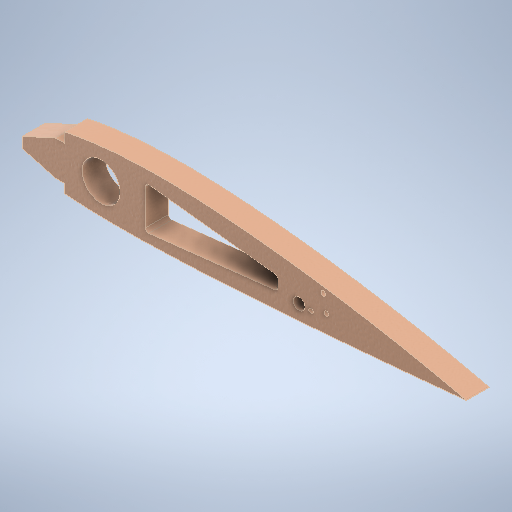
# Autodesk Inventor part: 2414 basic aerofoil
Saved by Autodesk Inventor 2025.1 (Build 291241000, 241)
## iProperties
Created: 2024-11-04
Part Number: 2414 basic aerofoil
Material: Polyurethane Foam
Document SubType Name: Modeling
Designer: johan
Density: 0.032 g/cm^3
Appearance: Coarse Textured - Umber
Author: johan
Autodesk Inventor part; units mm, degrees
ref_plane "YZ Plane" through (0, 0, 0) normal (1, 0, 0) x (0, 1, 0)
ref_plane "XZ Plane" through (0, 0, 0) normal (0, 1, 0) x (-1, 0, 0)
ref_plane "XY Plane" through (0, 0, 0) normal (0, 0, 1) x (1, 0, 0)
sketch "Sketch2" plane through (0, 0, 0) normal (0, 0, 1) x (1, 0, 0)
  spline S0 degree 5 poles (319.5633, 0.0573) (319.5622, 0.0645) (319.5873, 0.0852) (319.7357, 0.1422) (318.5514, 0.0989) (319.5116, 0.3205) (317.7694, 0.3117) (318.0865, 0.563) (316.6439, 0.6855) (316.0954, 0.948) (314.7794, 1.1779) (313.6787, 1.4773) (312.2394, 1.7863) (310.766, 2.136) (309.0996, 2.5093) (307.3242, 2.9134) (305.3998, 3.342) (303.349, 3.7975) (301.1634, 4.2757) (298.8504, 4.7782) (296.4091, 5.301) (293.8432, 5.8446) (291.1548, 6.4061) (288.3466, 6.9857) (285.4207, 7.5803) (282.3807, 8.1894) (279.2284, 8.8107) (275.968, 9.4437) (272.6016, 10.0865) (269.1329, 10.7361) (265.5656, 11.3942) (261.9019, 12.0551) (258.1469, 12.7207) (254.3029, 13.3883) (250.3742, 14.0555) (246.3647, 14.7217) (242.2776, 15.3854) (238.118, 16.0441) (233.8887, 16.6979) (229.5952, 17.3434) (225.2402, 17.981) (220.8297, 18.6074) (216.3658, 19.2226) (211.8552, 19.8242) (207.3009, 20.4107) (202.7077, 20.9813) (198.0804, 21.5339) (193.4232, 22.0679) (188.7413, 22.58) (184.0389, 23.0713) (179.321, 23.5382) (174.592, 23.982) (169.8567, 24.3971) (165.1201, 24.7874) (160.3872, 25.1472) (155.6604, 25.4776) (150.948, 25.7772) (146.2454, 26.0449) (141.5744, 26.278) (136.9015, 26.4795) (132.2479, 26.6311) (127.6319, 26.7393) (123.054, 26.7999) (118.5202, 26.8147) (114.0397, 26.7815) (109.6094, 26.7031) (105.2517, 26.5723) (100.9331, 26.4088) (96.7495, 26.1663) (92.5147, 25.9483) (88.6376, 25.5343) (84.2302, 25.3974) (81.2071, 24.5612) (76.5297, 24.5259) (73.18, 23.8676) (69.3619, 23.413) (65.9721, 22.8018) (62.3454, 22.244) (59.4319, 21.514) (55.4307, 21.0148) (53.2464, 20.1084) (49.5889, 19.537) (47.2944, 18.6473) (44.3884, 17.909) (41.914, 17.071) (39.4431, 16.2394) (37.1538, 15.3738) (34.9769, 14.4941) (32.9455, 13.5944) (31.0501, 12.6807) (29.296, 11.7542) (27.6838, 10.8151) (26.2147, 9.8673) (24.8899, 8.9103) (23.7091, 7.9466) (22.6766, 6.9761) (21.7838, 6.0003) (21.0519, 5.0188) (20.4402, 4.0317) (20.0369, 3.0394) (19.6679, 2.0412) (19.7059, 1.0482) (19.3667, 0.0428) (19.9014, -0.9137) (20.0594, -1.8759) (20.6154, -2.7916) (21.2041, -3.6802) (21.9915, -4.5317) (22.8926, -5.3516) (23.9468, -6.1384) (25.1324, -6.8944) (26.4586, -7.6188) (27.9182, -8.3124) (29.5137, -8.9751) (31.2408, -9.6071) (33.0997, -10.2067) (35.0892, -10.7758) (37.2002, -11.3131) (39.4562, -11.8174) (41.7927, -12.2939) (44.3651, -12.7275) (46.7744, -13.1584) (50.0005, -13.481) (52.1533, -13.8927) (55.9371, -14.1294) (58.2153, -14.4717) (61.732, -14.6854) (64.8012, -14.9153) (68.2287, -15.092) (71.6338, -15.2498) (75.1915, -15.3722) (78.8138, -15.4692) (82.5326, -15.5359) (86.3291, -15.5764) (90.2061, -15.5901) (94.1575, -15.5787) (98.1812, -15.5438) (102.2727, -15.4851) (106.4286, -15.4059) (110.6456, -15.3062) (114.9188, -15.1867) (119.2459, -15.0512) (123.6218, -14.8988) (128.0442, -14.7319) (132.5111, -14.552) (137.0141, -14.3592) (141.5621, -14.1606) (146.1675, -13.9403) (150.787, -13.7052) (155.434, -13.4523) (160.0951, -13.1857) (164.7676, -12.9046) (169.4465, -12.6129) (174.1261, -12.3082) (178.8033, -11.9955) (183.4722, -11.6727) (188.1294, -11.3426) (192.7696, -11.0072) (197.3886, -10.6641) (201.9818, -10.3188) (206.5448, -9.9678) (211.0728, -9.6157) (215.5623, -9.2611) (220.0069, -8.9047) (224.4048, -8.5497) (228.7492, -8.193) (233.0373, -7.8393) (237.2647, -7.4865) (241.4259, -7.1353) (245.5189, -6.7884) (249.5374, -6.4441) (253.4791, -6.104) (257.3389, -5.7683) (261.1136, -5.4376) (264.7987, -5.113) (268.3914, -4.7937) (271.8871, -4.4807) (275.2826, -4.1749) (278.5752, -3.8759) (281.7596, -3.585) (284.8354, -3.3021) (287.7962, -3.0278) (290.6419, -2.763) (293.3673, -2.5063) (295.9711, -2.2616) (298.4499, -2.0246) (300.8007, -1.801) (303.0232, -1.5859) (305.1102, -1.385) (307.0698, -1.1939) (308.8781, -1.0169) (310.5784, -0.8499) (312.0781, -0.7003) (313.5527, -0.5569) (314.6651, -0.4406) (316.0303, -0.3144) (316.5535, -0.2432) (318.0889, -0.1199) (317.6732, -0.1146) (319.5611, 0.0154) (318.488, -0.03) (319.7124, 0.0524) (319.5915, 0.0431) (319.5644, 0.0506) (319.5633, 0.0573) knots 0 0 0 0 0 0 0.001187 0.002346 0.003989 0.006081 0.008474 0.011129 0.014019 0.017125 0.020431 0.023922 0.027589 0.03142 0.035408 0.039543 0.04382 0.048231 0.05277 0.057431 0.062209 0.067099 0.072096 0.077195 0.082391 0.087681 0.09306 0.098523 0.104068 0.10969 0.115384 0.121149 0.126979 0.132871 0.138822 0.144829 0.150887 0.156993 0.163144 0.169337 0.175568 0.181834 0.188131 0.194457 0.200808 0.207181 0.213572 0.219979 0.226398 0.232826 0.239259 0.245695 0.252131 0.258563 0.264988 0.271403 0.277808 0.284202 0.290583 0.296947 0.303291 0.309608 0.315893 0.322143 0.328354 0.334523 0.340648 0.346723 0.352747 0.358657 0.364567 0.370414 0.376198 0.381913 0.387616 0.393187 0.398728 0.404136 0.40949 0.414723 0.419864 0.42486 0.429808 0.434623 0.439363 0.443992 0.448508 0.452906 0.457184 0.461338 0.465365 0.469264 0.473032 0.47667 0.480179 0.483564 0.486831 0.489993 0.493064 0.496069 0.499033 0.501972 0.504912 0.507875 0.510883 0.513952 0.517109 0.52037 0.523745 0.527242 0.530864 0.534612 0.538487 0.542486 0.546608 0.55085 0.555208 0.559679 0.564259 0.568979 0.573768 0.578707 0.583689 0.588762 0.59389 0.599137 0.604414 0.609823 0.615307 0.620863 0.626488 0.632178 0.63793 0.643742 0.64961 0.655531 0.661502 0.667521 0.673583 0.679687 0.685829 0.692006 0.698215 0.704456 0.710729 0.717031 0.723359 0.72971 0.736079 0.742458 0.748845 0.755237 0.76163 0.768021 0.774408 0.780786 0.787154 0.793507 0.799843 0.806158 0.812449 0.818713 0.824947 0.831148 0.837311 0.843434 0.849514 0.855546 0.861529 0.867457 0.873328 0.879138 0.884884 0.890561 0.896166 0.901696 0.907146 0.912512 0.91779 0.922975 0.928065 0.933053 0.937935 0.942706 0.947361 0.951895 0.956301 0.960574 0.964706 0.968691 0.97252 0.976185 0.979675 0.982979 0.986084 0.988974 0.991629 0.994021 0.996112 0.997735 0.998873 1 1 1 1 1 1
  circle A0 centre (79.5135, 4.5678) radius 12.4155
  line L0 (79.5135, 4.5678) -> (79.5135, 24.6083) construction
  circle A1 centre (209.5633, 0.0573) radius 3.786
  line L1 (319.5633, 0.0573) -> (219.5633, 0.0573) construction
  line L2 (27.919, 4.5057) -> (27.919, -2.4943)
  line L3 (19.627, 1.0326) -> (319.5633, 0.0573) construction
  line L4 (49.7105, 14.4213) -> (55.6079, 14.4213)
  line L5 (49.7104, -8.4915) -> (55.6078, -8.4915)
  line L6 (27.919, 4.5057) -> (49.7105, 14.4213)
  line L7 (27.919, -2.4943) -> (49.7104, -8.4915)
  line L8 (55.6079, 14.4213) -> (55.6079, 20.8726)
  line L9 (55.6078, -8.4915) -> (55.6078, -14.1513)
  line L10 (108.6496, 16.3299) -> (108.6496, -7.1942)
  line L11 (110.8735, -9.1817) -> (193.8736, 0.1678)
  line L12 (195.6498, 2.1552) -> (195.6498, 6.9805)
  line L13 (193.8736, 8.9679) -> (110.8735, 18.3173)
  arc A2 (110.8735, 18.3173) -> (108.6496, 16.3299) centre (110.6496, 16.3299) ccw
  arc A3 (108.6496, -7.1942) -> (110.8735, -9.1817) centre (110.6496, -7.1942) ccw
  arc A4 (193.8736, 0.1678) -> (195.6498, 2.1552) centre (193.6498, 2.1552) ccw
  arc A5 (195.6498, 6.9805) -> (193.8736, 8.9679) centre (193.6498, 6.9805) ccw
  circle A6 centre (227.5633, 3.4733) radius 1.5
  circle A7 centre (217.5082, 0.0573) radius 1.5
  circle A8 centre (225.5082, 13.9137) radius 1.5
  line L14 (227.5633, 3.4733) -> (254.2882, 3.4733) construction
  line L15 (227.5633, 3.4733) -> (184.262, 28.4733) construction
  line L16 (217.5082, 0.0573) -> (225.5082, 13.9137) construction
  point P0 (0, 0)
  point P1 (319.3573, 0.1272)
  point P2 (318.9918, 0.2142)
  point P3 (318.4802, 0.3354)
  point P4 (317.8238, 0.4911)
  point P5 (317.0222, 0.6801)
  point P6 (316.0769, 0.9024)
  point P7 (314.9885, 1.1568)
  point P8 (313.7582, 1.443)
  point P9 (312.3866, 1.7598)
  point P10 (310.8752, 2.1063)
  point P11 (309.2258, 2.4819)
  point P12 (307.4393, 2.8854)
  point P13 (305.5178, 3.3153)
  point P14 (303.4628, 3.7707)
  point P15 (301.2764, 4.2501)
  point P16 (298.9607, 4.7526)
  point P17 (296.5175, 5.2764)
  point P18 (293.9492, 5.8203)
  point P19 (291.2585, 6.3828)
  point P20 (288.4478, 6.9627)
  point P21 (285.5195, 7.5582)
  point P22 (282.4766, 8.1678)
  point P23 (279.3218, 8.79)
  point P24 (276.0584, 9.4236)
  point P25 (272.6891, 10.0668)
  point P26 (269.2175, 10.7178)
  point P27 (265.6469, 11.3757)
  point P28 (261.9803, 12.0381)
  point P29 (258.2219, 12.7041)
  point P30 (254.3747, 13.3722)
  point P31 (250.4426, 14.0403)
  point P32 (246.4295, 14.7072)
  point P33 (242.339, 15.3714)
  point P34 (238.1756, 16.0311)
  point P35 (233.9428, 16.6851)
  point P36 (229.6454, 17.3316)
  point P37 (225.2869, 17.9694)
  point P38 (220.8723, 18.5967)
  point P39 (216.4049, 19.2123)
  point P40 (211.8901, 19.8144)
  point P41 (207.332, 20.4015)
  point P42 (202.7347, 20.9724)
  point P43 (198.1034, 21.5256)
  point P44 (193.4423, 22.0596)
  point P45 (188.7563, 22.5726)
  point P46 (184.0499, 23.0637)
  point P47 (179.3279, 23.5314)
  point P48 (174.5948, 23.9745)
  point P49 (169.8554, 24.3909)
  point P50 (165.1148, 24.7803)
  point P51 (160.3775, 25.1406)
  point P52 (155.6479, 25.4709)
  point P53 (150.9316, 25.7703)
  point P54 (146.233, 26.0373)
  point P55 (141.557, 26.2707)
  point P56 (136.882, 26.4681)
  point P57 (132.2209, 26.6211)
  point P58 (127.5964, 26.7282)
  point P59 (123.0133, 26.7888)
  point P60 (118.4761, 26.8026)
  point P61 (113.9902, 26.7693)
  point P62 (109.5601, 26.6886)
  point P63 (105.191, 26.5611)
  point P64 (100.8866, 26.3866)
  point P65 (96.6524, 26.1647)
  point P66 (92.4927, 25.8975)
  point P67 (88.4121, 25.5832)
  point P68 (84.4152, 25.2282)
  point P69 (80.9052, 24.7441)
  point P70 (76.6873, 24.3761)
  point P71 (72.9635, 23.8905)
  point P72 (69.3402, 23.3611)
  point P73 (65.8208, 22.7938)
  point P74 (62.4086, 22.1883)
  point P75 (59.107, 21.5464)
  point P76 (52.8493, 20.1606)
  point P77 (49.7105, 19.4213)
  point P78 (47.0737, 18.6507)
  point P79 (44.3741, 17.8542)
  point P80 (41.8034, 17.0322)
  point P81 (39.3638, 16.1874)
  point P82 (37.0583, 15.3213)
  point P83 (34.8884, 14.4363)
  point P84 (32.8568, 13.534)
  point P85 (30.965, 12.6166)
  point P86 (29.2145, 11.686)
  point P87 (27.6071, 10.7437)
  point P88 (26.1443, 9.7921)
  point P89 (24.8269, 8.8324)
  point P90 (23.6566, 7.8664)
  point P91 (22.6336, 6.8953)
  point P92 (21.7591, 5.9209)
  point P93 (21.0334, 4.9441)
  point P94 (20.4571, 3.9661)
  point P95 (20.0308, 2.9875)
  point P96 (19.7539, 2.0098)
  point P97 (19.5632, 0.0573)
  point P98 (19.8205, -0.9033)
  point P99 (20.1376, -1.8357)
  point P100 (20.6002, -2.7402)
  point P101 (21.208, -3.6159)
  point P102 (21.9598, -4.4628)
  point P103 (22.8544, -5.2806)
  point P104 (23.8909, -6.069)
  point P105 (25.0681, -6.8277)
  point P106 (26.3846, -7.5561)
  point P107 (27.8384, -8.2539)
  point P108 (29.4284, -8.9211)
  point P109 (31.1522, -9.5571)
  point P110 (33.0086, -10.1613)
  point P111 (34.9949, -10.734)
  point P112 (37.1093, -11.2746)
  point P113 (39.3497, -11.7828)
  point P114 (41.7134, -12.2586)
  point P115 (44.198, -12.702)
  point P116 (46.8014, -13.1127)
  point P117 (49.7104, -13.4915)
  point P118 (52.3532, -13.8357)
  point P119 (58.3469, -14.4294)
  point P120 (61.5023, -14.6781)
  point P121 (64.7591, -14.8953)
  point P122 (68.1149, -15.0813)
  point P123 (71.5661, -15.237)
  point P124 (75.1094, -15.3627)
  point P125 (78.7418, -15.4596)
  point P126 (82.46, -15.528)
  point P127 (86.2607, -15.5691)
  point P128 (90.14, -15.5838)
  point P129 (94.0946, -15.5733)
  point P130 (98.1212, -15.5388)
  point P131 (102.2159, -15.4812)
  point P132 (106.3751, -15.4023)
  point P133 (110.5952, -15.303)
  point P134 (114.872, -15.1845)
  point P135 (119.2022, -15.0489)
  point P136 (123.5813, -14.8971)
  point P137 (128.006, -14.7306)
  point P138 (132.4718, -14.5509)
  point P139 (136.9748, -14.3598)
  point P140 (141.5285, -14.1576)
  point P141 (146.1365, -13.9383)
  point P142 (150.7679, -13.7022)
  point P143 (155.4191, -13.4499)
  point P144 (160.0853, -13.1829)
  point P145 (164.7617, -12.9024)
  point P146 (169.4444, -12.6099)
  point P147 (174.1283, -12.306)
  point P148 (178.8092, -11.9925)
  point P149 (183.4823, -11.67)
  point P150 (188.1434, -11.34)
  point P151 (192.7877, -11.0037)
  point P152 (197.4106, -10.6614)
  point P153 (202.0079, -10.3149)
  point P154 (206.5747, -9.9645)
  point P155 (211.1069, -9.6117)
  point P156 (215.5999, -9.2568)
  point P157 (220.0489, -8.9007)
  point P158 (224.4503, -8.5446)
  point P159 (228.7987, -8.1885)
  point P160 (233.0906, -7.8339)
  point P161 (237.3214, -7.4808)
  point P162 (241.4866, -7.1298)
  point P163 (245.5828, -6.7821)
  point P164 (249.6052, -6.4377)
  point P165 (253.5502, -6.0972)
  point P166 (257.4136, -5.7612)
  point P167 (261.1915, -5.4303)
  point P168 (264.88, -5.1051)
  point P169 (268.4758, -4.7856)
  point P170 (271.9747, -4.4724)
  point P171 (275.3734, -4.1661)
  point P172 (278.6686, -3.867)
  point P173 (281.8564, -3.5757)
  point P174 (284.9344, -3.2925)
  point P175 (287.8984, -3.018)
  point P176 (290.7463, -2.7525)
  point P177 (293.4745, -2.4963)
  point P178 (296.0806, -2.2503)
  point P179 (298.5616, -2.0142)
  point P180 (300.9151, -1.7892)
  point P181 (303.1387, -1.575)
  point P182 (305.23, -1.3728)
  point P183 (307.1866, -1.1823)
  point P184 (309.007, -1.0041)
  point P185 (310.6885, -0.8385)
  point P186 (312.2302, -0.6861)
  point P187 (313.6297, -0.5472)
  point P188 (314.8861, -0.4221)
  point P189 (315.9976, -0.3108)
  point P190 (316.9636, -0.2139)
  point P191 (317.7826, -0.1314)
  point P192 (318.4537, -0.0636)
  point P193 (318.9766, -0.0108)
  point P194 (319.3503, 0.027)
  point P195 (319.5743, 0.0498)
  point P196 (27.919, 1.0057)
  point P197 (108.6496, 18.5678)
  point P198 (108.6496, -9.4322)
  point P199 (195.6498, 0.3678)
  dimension "d2" = 300.0001
  dimension "d18" = 7.572
  dimension "d19" = 110
  dimension "d22" = 100
  dimension "d23" = 7
  dimension "d24" = 5
  dimension "d25" = 5
  dimension "d30" = 28
  dimension "d31" = 8.4
  dimension "d34" = 2
  dimension "d37" = 24.831
  dimension "d44" = 3
  dimension "d45" = 92
  dimension "d46" = 3.416
  dimension "d49" = 3
  dimension "d50" = 3
  dimension "d51" = 50
  dimension "d52" = 150
  dimension "d53" = 16
  dimension "d54" = 7
  dimension "d58" = 59.8865
  constraints: 34 end point, 9 centre point, 9 point on line, 8 point on circle, 8 tangent, 4 vertical, 3 equal radius, 3 midpoint, 2 horizontal, 2 horizontal alignment, 1 parallel, 1 perpendicular, 201 other
  measures "d2" distance of L1.start point (19.563, 0.057)
  measures "d18" diameter of A1
  measures "d19" distance of L1.start A1.centre
  measures "d22" distance of L1.start L1.end
  measures "d23" distance of L2.start L2.end
  measures "d24" distance from line of point (49.71, 19.421) L4
  measures "d25" distance from line of point (49.71, -13.491) L5
  measures "d30" distance of point (108.65, 18.568) point (108.65, -9.432)
  measures "d31" distance of point (195.65, 0.368) point (195.65, 8.768)
  measures "d34" radius of A2
  measures "d37" diameter of A0
  measures "d44" diameter of A6
  measures "d45" horizontal distance of L1.start L14.start
  measures "d46" distance from line of L1 L14.start
  measures "d49" diameter of A7
  measures "d50" diameter of A8
  measures "d51" distance of L14.start L15.end
  measures "d52" angle of L15 L14
  measures "d53" distance of L16.start L16.end
  measures "d54" distance from line of L16 L14.start
  measures "d58" horizontal distance of L3.start L0.start
extrude "Extrusion8" add sketch "Sketch2" along normal blind 15 contours S0 L9 L5 L7 L2 L6 L4 L8 picked at (144.7888, 17.9907)
body "Solid8"
